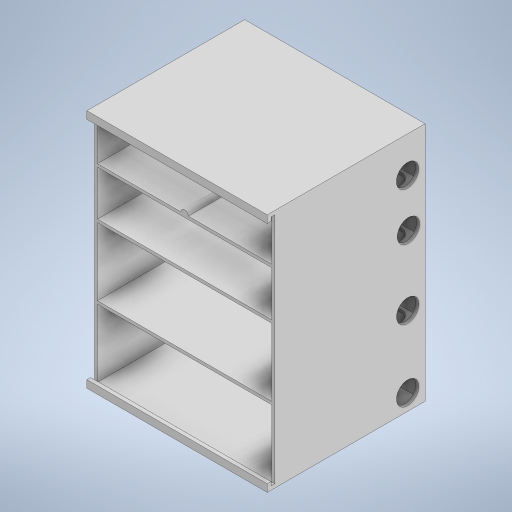
# Autodesk Inventor part: Shelf
Saved by Autodesk Inventor 2024 (Build 280153000, 153)
## iProperties
Created: 2023-10-02
Part Number: Shelf
Material: Generic
Document SubType Name: Modeling
Designer: vegaj
Density: 1 g/cm^3
Appearance: Default
Author: vegaj
Autodesk Inventor part; units mm, degrees
ref_plane "YZ Plane" through (0, 0, 0) normal (1, 0, 0) x (0, 1, 0)
ref_plane "XZ Plane" through (0, 0, 0) normal (0, 1, 0) x (-1, 0, 0)
ref_plane "XY Plane" through (0, 0, 0) normal (0, 0, 1) x (1, 0, 0)
sketch "Sketch2" plane through (0, 0, 0) normal (0, 1, 0) x (-1, 0, 0)
  line L0 (0, 0) -> (152.4, 0)
  line L1 (152.4, 0) -> (152.4, -127)
  line L2 (152.4, -127) -> (0, -127)
  line L3 (0, -127) -> (0, 0)
  dimension "d2" = 152.4
  dimension "d3" = 127
  constraints: 8 end point, 2 parallel, 1 horizontal, 1 perpendicular
  measures "d2" distance of L1.end L2.end
  measures "d3" distance of L0.end L1.end
extrude "Extrusion1" add sketch "Sketch2" along normal blind 2.54
sketch "Sketch3" plane through (0, 0, 0) normal (1, 0, 0) x (0, 0, -1)
  line L0 (127, 2.54) -> (0, 2.54) projected
  line L1 (0, 2.54) -> (127, 2.54)
  line L2 (127, 2.54) -> (127, 203.2)
  line L3 (127, 203.2) -> (0, 203.2)
  line L4 (0, 203.2) -> (0, 2.54)
  point P0 (0, 0)
  dimension "d6" = 127
  dimension "d7" = 200.66
  constraints: 8 end point, 2 parallel, 1 horizontal, 1 perpendicular
  measures "d6" distance of L3.end L2.end
  measures "d7" distance of L2.end L1.end
extrude "Extrusion2" add sketch "Sketch3" against normal blind 2.54
sketch "Sketch4" plane through (-152.4, 0, -127) normal (-1, 0, 0) x (0, 0, 1)
  line L0 (0, 2.54) -> (127, 2.54) projected
  line L1 (127, 0) -> (127, 203.2) projected
  line L2 (0, 2.54) -> (127, 2.54)
  line L3 (127, 2.54) -> (127, 203.2)
  line L4 (127, 203.2) -> (0, 203.2)
  line L5 (0, 203.2) -> (0, 2.54)
  constraints: 8 end point, 2 parallel, 1 horizontal, 1 perpendicular
extrude "Extrusion3" add sketch "Sketch4" against normal blind 2.54
sketch "Sketch5" plane through (0, 0, -127) normal (0, 0, -1) x (-1, 0, 0)
  line L0 (2.54, 2.54) -> (2.54, 203.2) projected
  line L1 (152.4, 203.2) -> (149.86, 203.2) projected
  line L2 (2.54, 2.54) -> (149.86, 2.54)
  line L3 (149.86, 2.54) -> (149.86, 203.2)
  line L4 (149.86, 203.2) -> (2.54, 203.2)
  line L5 (2.54, 203.2) -> (2.54, 2.54)
  point P0 (0, 0)
  constraints: 8 end point, 2 parallel, 1 horizontal, 1 perpendicular
extrude "Extrusion4" add sketch "Sketch5" against normal blind 2.54
sketch "Sketch6" plane through (-152.4, 203.2, 0) normal (0, 1, 0) x (1, 0, 0)
  line L0 (0, 0) -> (2.54, 0) projected
  line L1 (149.86, 124.46) -> (2.54, 124.46) projected
  line L2 (2.54, 0) -> (149.86, 0)
  line L3 (149.86, 0) -> (149.86, 124.46)
  line L4 (149.86, 124.46) -> (2.54, 124.46)
  line L5 (2.54, 124.46) -> (2.54, 0)
  point P0 (152.4, 0)
  constraints: 8 end point, 2 parallel, 1 horizontal, 1 perpendicular
extrude "Extrusion5" add sketch "Sketch6" against normal blind 2.54
sketch "Sketch7" plane through (-152.4, 0, 0) normal (0, 0, 1) x (1, 0, 0)
  line L0 (2.54, 200.66) -> (2.54, 2.54) projected
  line L1 (149.86, 200.66) -> (149.86, 2.54) projected
  line L2 (2.54, 59.69) -> (149.86, 59.69)
  line L3 (149.86, 59.69) -> (149.86, 62.23)
  line L4 (149.86, 62.23) -> (2.54, 62.23)
  line L5 (2.54, 62.23) -> (2.54, 59.69)
  line L6 (2.54, 119.38) -> (149.86, 119.38)
  line L7 (149.86, 119.38) -> (149.86, 121.92)
  line L8 (149.86, 121.92) -> (2.54, 121.92)
  line L9 (2.54, 121.92) -> (2.54, 119.38)
  line L10 (2.54, 160.02) -> (149.86, 160.02)
  line L11 (149.86, 160.02) -> (149.86, 162.56)
  line L12 (149.86, 162.56) -> (2.54, 162.56)
  line L13 (2.54, 162.56) -> (2.54, 160.02)
  dimension "d21" = 2.54
  dimension "d22" = 2.54
  dimension "d23" = 2.54
  constraints: 24 end point, 6 parallel, 6 point on line, 3 horizontal, 3 perpendicular
  measures "d21" distance of L3.end L2.end
  measures "d22" distance of L7.end L6.end
  measures "d23" distance of L11.end L10.end
extrude "Extrusion6" add sketch "Sketch7" against normal blind 126.365 contours L12 L1 L10 L0 | L8 L1 L6 L0 | L4 L1 L2 L0
sketch "Sketch8" plane through (0, 0, 0) normal (1, 0, 0) x (0, 0, -1)
  point P0 (0, 0)
  point P1 (112.1689, 172.8914)
  point P2 (112.9467, 132.1734)
  point P3 (112.3284, 73.8307)
  point P4 (112.2777, 13.6778)
hole "Hole1" at (0, 172.8914, -112.1689) at (0, 132.1734, -112.9467) at (0, 73.8307, -112.3284) at (0, 13.6778, -112.2777) direction (-1, 0, 0) diameter 19.05 depth 201.6125 tip angle 126
sketch "Sketch9" plane through (-149.86, 162.56, 0) normal (0, 1, 0) x (1, 0, 0)
  point P0 (149.86, 0)
  point P1 (11.1706, 112.6616)
  point P2 (134.449, 112.5332)
hole "Hole2" at (-15.411, 162.56, -112.5332) at (-138.6894, 162.56, -112.6616) direction (0, -1, 0) diameter 19.05 depth 149.225 tip angle 126
sketch "Sketch10" plane through (-152.4, 0, 0) normal (0, 0, 1) x (1, 0, 0)
  line L0 (149.86, 162.56) -> (2.54, 162.56) projected
  arc A0 (79.375, 162.56) -> (73.025, 162.56) centre (76.2, 162.56) ccw
  point P0 (152.4, 0)
  dimension "d40" = 6.35
  constraints: 2 point on circle, 2 point on line, 1 centre point, 1 midpoint
  measures "d40" diameter of A0
extrude "Extrusion7" add sketch "Sketch10" against normal blind 126.365
sketch "Sketch11" plane through (0, 0, 0) normal (1, 0, 0) x (0, 0, -1)
  line L0 (0, 0) -> (127, 0) projected
  line L1 (0, 0) -> (-6.35, 0)
  line L2 (-6.35, 0) -> (-6.35, 6.3374)
  line L3 (-6.35, 6.3374) -> (-3.175, 6.3374)
  line L4 (0, 6.3374) -> (0, 0)
  line L5 (0, 6.3374) -> (-3.175, 6.3374)
  line L6 (-3.175, 6.3374) -> (-3.175, 3.1687)
  line L7 (-3.175, 3.1687) -> (0, 3.1687)
  line L8 (0, 3.1687) -> (0, 6.3374)
  dimension "d43" = 6.35
  constraints: 16 end point, 4 parallel, 2 horizontal, 2 perpendicular
  measures "d43" distance of L2.end L4.start
extrude "Extrusion8" add sketch "Sketch11" against normal blind 152.4 contours L1 L2 L3 L6 L7 L4
sketch "Sketch13" plane through (0, 203.2, 0) normal (1, 0, 0) x (0, 0, -1)
  line L0 (0, -200.0313) -> (0, 0) projected
  line L1 (0, 0) -> (-6.35, 0)
  line L2 (-6.35, 0) -> (-6.35, -6.35)
  line L3 (-6.35, -6.35) -> (-3.175, -6.35)
  line L4 (0, -6.35) -> (0, 0)
  line L5 (0, -6.35) -> (-3.175, -6.35)
  line L6 (-3.175, -6.35) -> (-3.175, -3.175)
  line L7 (-3.175, -3.175) -> (0, -3.175)
  line L8 (0, -3.175) -> (0, -6.35)
  point P0 (0, -203.2)
  point P1 (0, -3.175)
  dimension "d50" = 6.35
  dimension "d51" = 6.35
  constraints: 16 end point, 4 parallel, 2 horizontal, 2 perpendicular
  measures "d50" distance of L4.start L2.end
  measures "d51" distance of L2.end L1.end
extrude "Extrusion10" add sketch "Sketch13" against normal blind 152.4 contours L7 L6 L3 L2 L1 L0
body "Solid1"
